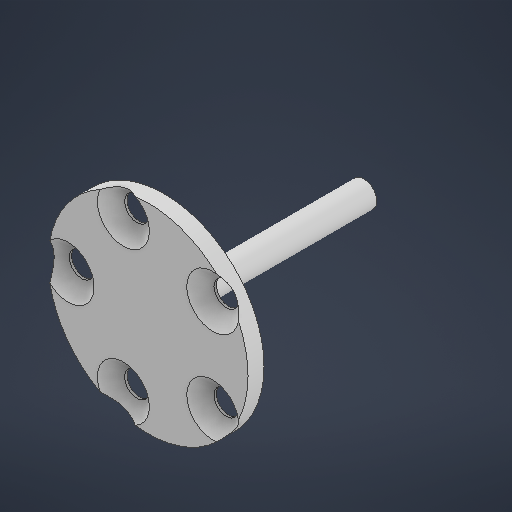
# Autodesk Inventor part: formadol
Saved by Autodesk Inventor 2026.2 (Build 302298010, 298A)
## iProperties
Created: 2026-05-11
Part Number: formadol
Material: Generic
Document SubType Name: Modeling
Designer: karol
Density: 1 g/cm^3
Appearance: Default
Author: karol
Autodesk Inventor part; units mm, degrees
ref_plane "YZ Plane" through (0, 0, 0) normal (1, 0, 0) x (0, 1, 0)
ref_plane "XZ Plane" through (0, 0, 0) normal (0, 1, 0) x (-1, 0, 0)
ref_plane "XY Plane" through (0, 0, 0) normal (0, 0, 1) x (1, 0, 0)
ref_plane "Work Plane1" through (14.6215, -13.2895, -4.736) normal (0, 0, 1) x (1, 0, 0)
sketch "Sketch1" plane through (14.6215, -13.2895, -4.736) normal (0, 0, 1) x (1, 0, 0)
  circle A0 centre (0, 0) radius 4 projected
  arc A1 (-1.3, -1.0954) -> (-1.3, 1.0954) centre (0, 0) ccw projected
  line L0 (-1.3, -1.0954) -> (-1.3, 1.0954) projected
  circle A2 centre (0, 0) radius 6
  circle A3 centre (0, 0) radius 12.5
  circle A4 centre (0, 0) radius 1.3331
  point P0 (-14.6215, 13.2895)
  dimension "d0" = 12
  dimension "d1" = 25
  constraints: 3 centre point, 3 coincident
  measures "d0" diameter of A2
  measures "d1" diameter of A3
extrude "Extrusion1" add sketch "Sketch1" along normal blind 2 contours A0 | L0 A4 A1 | A4 L0 | L0 A4 | A2 | A3
sketch "Sketch2" plane through (14.6215, -13.2895, -4.736) normal (0, 0, 1) x (1, 0, 0)
  circle A0 centre (0, 0) radius 4 projected
  arc A1 (-1.3, -1.0954) -> (-1.3, 1.0954) centre (0, 0) ccw projected
  line L0 (-1.3, -1.0954) -> (-1.3, 1.0954) projected
  circle A2 centre (0, 0) radius 6
  circle A3 centre (0, 0) radius 12.5
  circle A4 centre (-10, 0) radius 1.55
  circle A5 centre (-3.0902, -9.5106) radius 1.55
  circle A6 centre (8.0902, -5.8779) radius 1.55
  circle A7 centre (8.0902, 5.8779) radius 1.55
  circle A8 centre (-3.0902, 9.5106) radius 1.55
  point P0 (-14.6215, 13.2895)
  dimension "d4" = 12
  dimension "d5" = 25
  dimension "d6" = 3.1
  dimension "d7" = 10
  dimension "d10" = 360
  constraints: 7 centre point, 2 coincident, 11 other
  measures "d4" diameter of A2
  measures "d5" diameter of A3
  measures "d6" diameter of A4
  measures "d7" distance of A3.centre A4.centre
extrude "Extrusion2" cut sketch "Sketch2" along normal blind 22 contours A4 | A5 | A6 | A7 | A8
chamfer "Chamfer1" distance 1.7 angle 45 5 edges at (9.9813, -3.779, -2.736) (3.0715, -13.2895, -2.736) (21.1616, -7.4117, -2.736) (21.1616, -19.1674, -2.736) (9.9813, -22.8001, -2.736)
sketch "Sketch3" plane through (14.6215, -13.2895, -4.736) normal (0, 0, -1) x (-1, 0, 0)
  circle A0 centre (0, 0) radius 1.6
  line L0 (1.4, -0.7746) -> (1.4, 0.7746)
  point P0 (14.6215, 13.2895)
  point P1 (0.6764, 1.45)
  point P2 (-0.6764, 1.45)
  dimension "d17" = 3.2
  dimension "d21" = 1.4
  constraints: 4 point on circle, 2 end point, 1 centre point, 1 vertical, 1 other
  measures "d17" diameter of A0
  measures "d21" distance from line of A0.centre L0
extrude "Extrusion3" add sketch "Sketch3" along normal blind 25 contours L0 A0 picked at (0.3828, -0.3513)
body "Solid1"
